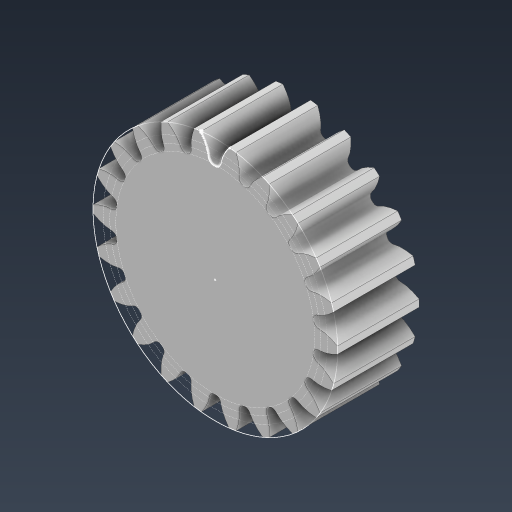
# Autodesk Inventor part: Деталь6
Saved by Autodesk Inventor 2023.2 (Build 272271030, 271C)
## iProperties
Created: 2025-12-05
Part Number: Деталь6
Material: Generic
Document SubType Name: Modeling
Designer: Олег Коноваленко
Density: 1 g/cm^3
Appearance: Default
Author: Олег Коноваленко
Autodesk Inventor part; units mm, degrees
ref_plane "YZ Plane" through (0, 0, 0) normal (1, 0, 0) x (0, 1, 0)
ref_plane "XZ Plane" through (0, 0, 0) normal (0, 1, 0) x (-1, 0, 0)
ref_plane "XY Plane" through (0, 0, 0) normal (0, 0, 1) x (1, 0, 0)
sketch "Sketch1" plane through (0, 0, 0) normal (0, 0, 1) x (1, 0, 0)
  spline S0 degree 3 poles (-2.7152, 23.8459) (-2.6479, 23.7553) (-2.5134, 23.574) (-2.3217, 23.2947) (-2.1382, 23.0101) (-1.9642, 22.7195) (-1.8005, 22.423) (-1.6483, 22.1204) (-1.5321, 21.8631) (-1.4465, 21.6542) (-1.3864, 21.4959) (-1.3307, 21.336) (-1.2799, 21.1744) (-1.2352, 21.0111) (-1.1833, 20.7912) (-1.1586, 20.5662) (-1.1094, 20.3746) (-1.077, 20.2665) (-1.0467, 20.1874) (-1.0142, 20.1092) (-0.9765, 20.0333) (-0.9338, 19.9601) (-0.8866, 19.8898) (-0.8341, 19.8233) (-0.7764, 19.7613) (-0.7139, 19.704) (-0.6461, 19.6532) (-0.5746, 19.6077) (-0.4986, 19.5699) (-0.4192, 19.5403) (-0.3376, 19.5175) (-0.254, 19.5032) (-0.1411, 19.4981) (0, 19.5013) (0.1411, 19.4981) (0.254, 19.5032) (0.3376, 19.5175) (0.4192, 19.5403) (0.4986, 19.5699) (0.5746, 19.6077) (0.6461, 19.6532) (0.7139, 19.704) (0.7764, 19.7613) (0.8341, 19.8233) (0.8866, 19.8898) (0.9338, 19.9601) (0.9765, 20.0333) (1.0142, 20.1092) (1.0467, 20.1874) (1.077, 20.2665) (1.1094, 20.3746) (1.1586, 20.5662) (1.1833, 20.7912) (1.2352, 21.0111) (1.2799, 21.1744) (1.3307, 21.336) (1.3864, 21.4959) (1.4465, 21.6542) (1.5321, 21.8631) (1.6483, 22.1204) (1.8005, 22.423) (1.9642, 22.7195) (2.1382, 23.0101) (2.3217, 23.2947) (2.5134, 23.574) (2.6479, 23.7553) (2.7152, 23.8459) knots 0 0 0 0 0.033863 0.067726 0.10159 0.135452 0.169315 0.203177 0.237039 0.253971 0.270903 0.287834 0.304766 0.321697 0.338628 0.372486 0.389413 0.397879 0.406344 0.414809 0.423275 0.431741 0.440206 0.448671 0.457135 0.465597 0.474059 0.482522 0.490988 0.49945 0.507913 0.516378 0.524841 0.541772 0.558704 0.567167 0.575632 0.584095 0.592557 0.601023 0.609486 0.617948 0.62641 0.634874 0.643339 0.651804 0.66027 0.668736 0.6772 0.685666 0.694132 0.711059 0.744917 0.761848 0.778779 0.795711 0.812642 0.829574 0.846506 0.880367 0.91423 0.948092 0.981955 1.015818 1.049682 1.083545 1.083545 1.083545 1.083545
  circle A0 centre (0, 0) radius 19.5 construction
  circle A1 centre (0, 0) radius 20.6732 construction
  circle A2 centre (0, 0) radius 22 construction
  circle A3 centre (0, 0) radius 24
  point P0 (-2.5151, 23.5728)
  point P1 (-2.3231, 23.2938)
  point P2 (-2.1398, 23.0091)
  point P3 (-1.9659, 22.7185)
  point P4 (-1.8024, 22.4219)
  point P5 (-1.6504, 22.1194)
  point P6 (-1.5113, 21.8106)
  point P7 (-1.4472, 21.6539)
  point P8 (-1.3871, 21.4956)
  point P9 (-1.3315, 21.3357)
  point P10 (-1.2809, 21.1741)
  point P11 (-1.2362, 21.0108)
  point P12 (-1.1986, 20.8458)
  point P13 (-1.1419, 20.5119)
  point P14 (-1.101, 20.3477)
  point P15 (-1.076, 20.2668)
  point P16 (-1.0463, 20.1875)
  point P17 (-1.0133, 20.1096)
  point P18 (-0.9757, 20.0338)
  point P19 (-0.9331, 19.9606)
  point P20 (-0.8857, 19.8904)
  point P21 (-0.8332, 19.824)
  point P22 (-0.7756, 19.7621)
  point P23 (-0.713, 19.7051)
  point P24 (-0.6455, 19.6541)
  point P25 (-0.5739, 19.609)
  point P26 (-0.498, 19.5713)
  point P27 (-0.4189, 19.5415)
  point P28 (-0.3373, 19.5189)
  point P29 (-0.2538, 19.5049)
  point P30 (-0.1693, 19.5)
  point P31 (0, 19.5)
  point P32 (0.1693, 19.5)
  point P33 (0.2538, 19.5049)
  point P34 (0.3373, 19.5189)
  point P35 (0.4189, 19.5415)
  point P36 (0.498, 19.5713)
  point P37 (0.5739, 19.609)
  point P38 (0.6455, 19.6541)
  point P39 (0.713, 19.7051)
  point P40 (0.7756, 19.7621)
  point P41 (0.8332, 19.824)
  point P42 (0.8857, 19.8904)
  point P43 (0.9331, 19.9606)
  point P44 (0.9757, 20.0338)
  point P45 (1.0133, 20.1096)
  point P46 (1.0463, 20.1875)
  point P47 (1.076, 20.2668)
  point P48 (1.101, 20.3477)
  point P49 (1.1419, 20.5119)
  point P50 (1.1986, 20.8458)
  point P51 (1.2362, 21.0108)
  point P52 (1.2809, 21.1741)
  point P53 (1.3315, 21.3357)
  point P54 (1.3871, 21.4956)
  point P55 (1.4472, 21.6539)
  point P56 (1.5113, 21.8106)
  point P57 (1.6504, 22.1194)
  point P58 (1.8024, 22.4219)
  point P59 (1.9659, 22.7185)
  point P60 (2.1398, 23.0091)
  point P61 (2.3231, 23.2938)
  point P62 (2.5151, 23.5728)
  constraints: 4 centre point, 2 point on circle, 135 other
extrude "Выдавливание1" add sketch "Sketch1" against normal blind 16
extrude "Выдавливание2" cut sketch "Sketch1" against normal through all contours A3 S0 picked at (-0.4326, 22.5744)
pattern_circular "Круговой массив1" count 22 over 360 about axis through (0, 0, 0) along (0, 0, -1) of "Выдавливание2"
equation "\"d0\" = Ширина_грани"
equation "\"Модуль\" = 2"
equation "\"Угол_зацепления\" = 20deg"
equation "\"Зазор_профиля_зуба\" = 0.25"
equation "\"Радиус_закругления_зуба\" = 0.35"
equation "\"Диаметр_головки\" = 48"
equation "\"Диаметр_впадин\" = 39"
equation "\"Основной_диаметр\" = 41.34648"
equation "\"Средний_диаметр\" = 44"
equation "\"Ширина_грани\" = 16"
equation "\"Коэффициент_смещения\" = 0"
equation "\"Изменение_высоты_головки_зуба\" = 0"
equation "\"Окружной_шаг\" = 6.283185"
equation "\"Общий_сдвиг_инструмента\" = 0"
equation "\"Внутренний\" = 0"
